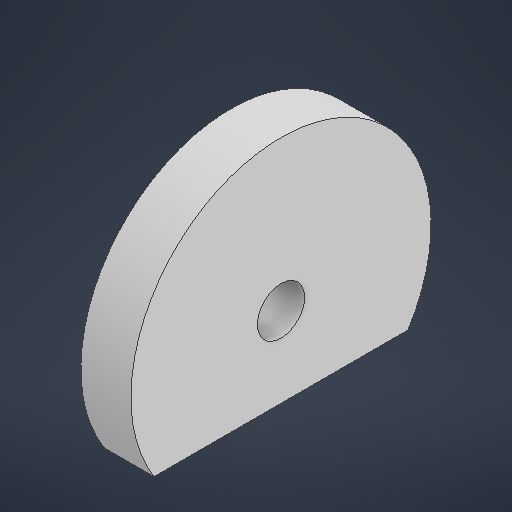
# Autodesk Inventor part: WheelConnector
Saved by Autodesk Inventor 2026.1 (Build 301233000, 233)
## iProperties
Created: 2026-07-03
Part Number: WheelConnector
Material: Generic
Document SubType Name: Modeling
Designer: Kasi Pusuluri
Density: 1 g/cm^3
Appearance: Default
Author: Kasi Pusuluri
Autodesk Inventor part; units mm, degrees
ref_plane "YZ Plane" through (0, 0, 0) normal (1, 0, 0) x (0, 1, 0)
ref_plane "XZ Plane" through (0, 0, 0) normal (0, 1, 0) x (-1, 0, 0)
ref_plane "XY Plane" through (0, 0, 0) normal (0, 0, 1) x (1, 0, 0)
sketch "Sketch1" plane through (0, 0, 0) normal (1, 0, 0) x (0, 1, 0)
  circle A0 centre (0, 0) radius 9.525
  line L0 (0, 10.3132) -> (0, -10.4019)
  line L1 (0, 9.525) -> (-5.08, 9.525)
  line L2 (-5.08, 9.525) -> (-5.08, -9.525)
  line L3 (-5.08, -9.525) -> (0, -9.525)
  line L4 (0, -9.525) -> (0, 9.525)
  circle A1 centre (0, 0) radius 1.5
  point P0 (-5.08, 8.0572)
  point P1 (-5.08, -8.0572)
  dimension "d0" = 19.05
  dimension "d1" = 3
  dimension "d2" = 5.08
  constraints: 10 end point, 2 coincident, 2 parallel, 1 centre point, 1 horizontal, 1 perpendicular, 1 point on line, 1 vertical, 3 other
  measures "d1" diameter of A1
  measures "d2" distance of L2.end L3.end
extrude "Extrusion1" add sketch "Sketch1" along normal blind 3.175 contours A0 L0 A1 | L0 A1 A0 L2
body "Solid1"
